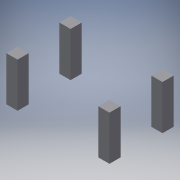
# Autodesk Inventor part: Z bars
Saved by Autodesk Inventor 2018.1 (Build 221171000, 171)
## iProperties
Created: 2024-06-06
Part Number: Z bars
Material: Generic
Document SubType Name: Modeling
Designer: Enrico
Density: 1 g/cm^3
Appearance: Default
Author: Enrico
Autodesk Inventor part; units mm, degrees
ref_plane "YZ Plane" through (0, 0, 0) normal (1, 0, 0) x (0, 1, 0)
ref_plane "XZ Plane" through (0, 0, 0) normal (0, 1, 0) x (-1, 0, 0)
ref_plane "XY Plane" through (0, 0, 0) normal (0, 0, 1) x (1, 0, 0)
sketch "Sketch1" plane through (0, 0, 0) normal (0, 0, 1) x (1, 0, 0)
  line L0 (371.8, 0) -> (0, 0) construction
  line L1 (0, 0) -> (0, 40) construction
  line L2 (371.8, 40) -> (0, 40) construction
  line L3 (371.8, 0) -> (371.8, 40) construction
  line L4 (0, 0) -> (40, 0) construction
  line L5 (40, 0) -> (40, 40)
  line L6 (40, 40) -> (0, 40) construction
  line L7 (0, 40) -> (0, 0) construction
  line L8 (185.9, 0) -> (185.9, 231.5) construction
  line L9 (371.8, 231.5) -> (0, 231.5) construction
  line L10 (371.8, 191.4) -> (371.8, 40.1) construction
  line L11 (0, 191.4) -> (0, 40.1) construction
  line L12 (371.8, 115.75) -> (0, 115.75) construction
  line L13 (40, 40) -> (0, 40)
  line L14 (0, 40) -> (0, 0)
  line L15 (0, 0) -> (40, 0)
  line L16 (40, 0) -> (40, 40)
  line L17 (0, 231.5) -> (40, 231.5)
  line L18 (40, 231.5) -> (40, 191.5)
  line L19 (40, 191.5) -> (0, 191.5)
  line L20 (0, 191.5) -> (0, 231.5)
  line L21 (371.8, 0) -> (371.8, 40) construction
  line L22 (371.8, 0) -> (331.8, 0) construction
  line L23 (331.8, 0) -> (331.8, 40)
  line L24 (331.8, 40) -> (371.8, 40) construction
  line L25 (371.8, 40) -> (371.8, 0) construction
  line L26 (371.8, 191.4) -> (371.8, 40.1) construction
  line L27 (331.8, 40) -> (371.8, 40)
  line L28 (371.8, 40) -> (371.8, 0)
  line L29 (371.8, 0) -> (331.8, 0)
  line L30 (331.8, 0) -> (331.8, 40)
  line L31 (371.8, 231.5) -> (331.8, 231.5)
  line L32 (331.8, 231.5) -> (331.8, 191.5)
  line L33 (331.8, 191.5) -> (371.8, 191.5)
  line L34 (371.8, 191.5) -> (371.8, 231.5)
  dimension "d0" = 40
  dimension "d1" = 40
  dimension "d2" = 40
  constraints: 56 end point, 9 symmetric about line, 6 parallel, 4 midpoint, 3 horizontal, 3 perpendicular, 1 point on line, 1 vertical
  measures "d0" distance between parallel lines of L1 L5
  measures "d1" distance between parallel lines of L20 L18
  measures "d2" distance between parallel lines of L17 L19
ref_plane "Work Plane1" through (-749.4514, -2, 159.9) normal (0, 0, -1) x (0, 1, 0)
ref_plane "Work Plane2" through (0, 0, 259.9) normal (0, 0, -1) x (0, 1, 0)
ref_plane "Work Plane3" through (0, 0, 159.9) normal (0, 0, -1) x (0, 1, 0)
ref_plane "Work Plane4" through (0, 0, 209.9) normal (0, 0, -1) x (0, 1, 0)
extrude "Extrusion1" add sketch "Sketch1" along normal up to surface (209.9 mm away)
body "Solid1"
